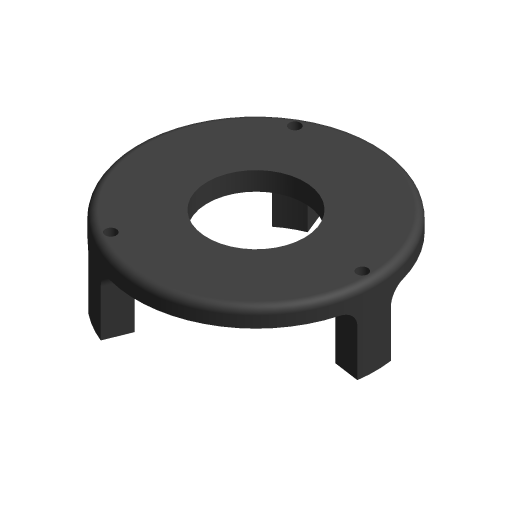
# Autodesk Inventor part: Engine retention
Saved by Autodesk Inventor 2024 (Build 280153000, 153)
## iProperties
Part Number: Engine retention
Material: Generic
Document SubType Name: Modeling
Designer: Jamie
Appearance: Default
Author: Jamie
Autodesk Inventor part; units mm, degrees
ref_plane "YZ Plane" through (0, 0, 0) normal (1, 0, 0) x (0, 1, 0)
ref_plane "XZ Plane" through (0, 0, 0) normal (0, 1, 0) x (-1, 0, 0)
ref_plane "XY Plane" through (0, 0, 0) normal (0, 0, 1) x (1, 0, 0)
sketch "Sketch1" plane through (0, 0, 0) normal (0, 1, 0) x (-1, 0, 0)
  circle A0 centre (0, 0) radius 25
  circle A1 centre (0, 0) radius 32
  dimension "d0" = 50
  dimension "d1" = 64
  constraints: 2 centre point, 2 coincident
  measures "d0" diameter of A0
  measures "d1" diameter of A1
extrude "Extrusion1" add sketch "Sketch1" along normal blind 16.5
sketch "Sketch2" plane through (0, 16.5, 0) normal (0, 1, 0) x (1, 0, 0)
  circle A0 centre (0, 0) radius 13
  circle A1 centre (0, 0) radius 32
  dimension "d4" = 26
  constraints: 2 centre point, 2 coincident
  measures "d4" diameter of A0
extrude "Extrusion2" add sketch "Sketch2" along normal blind 5
sketch "Sketch4" plane through (0, 0, 0) normal (0, -1, 0) x (1, 0, 0)
  circle A0 centre (28.5, 0) radius 1.5
  circle A1 centre (0, 0) radius 25 projected
  circle A2 centre (0, 0) radius 32 projected
  dimension "d7" = 3
  dimension "d9" = 28.5
  constraints: 1 centre point
  measures "d7" diameter of A0
  measures "d9" distance of A2.centre A0.centre
extrude "Extrusion3" cut sketch "Sketch4" against normal through all contours A0
pattern_circular "Circular Pattern1" count 3 over 360 about axis through (0, 0, 0) along (0, 1, 0) of "Extrusion3"
sketch "Sketch5" plane through (0, 0, 0) normal (0, -1, 0) x (1, 0, 0)
  line L0 (0, 0) -> (36.13577, -5.122389)
  line L1 (36.13577, -5.122389) -> (37.678755, -25.438365)
  line L2 (37.678755, -25.438365) -> (-15.629216, -38.816532)
  circle A0 centre (0, 0) radius 32
  line L3 (-15.629216, -38.816532) -> (0, 0)
  circle A1 centre (28.5, 0) radius 1.5
  circle A2 centre (-14.25, -24.681724) radius 1.5
  point P0 (-11.952112, -29.684121)
  point P1 (31.683259, -4.491228)
  dimension "d15" = 4
  dimension "d22" = 4
  constraints: 8 end point
  measures "d15" distance from line of A1.centre L0
  measures "d22" distance from line of A2.centre L3
extrude "Extrusion4" cut sketch "Sketch5" against normal blind 16.5 contours L0 A0 L3 picked at (20.515863, -5.328549)
pattern_circular "Circular Pattern2" count 3 over 360 about axis through (0, 16.5, 0) along (0, 1, 0) of "Extrusion4"
fillet "Fillet1" radius 4 6 edges at (28.2179, 16.5, -4) (-10.6448, 16.5, -26.4374) (-17.5731, 16.5, -22.4374) (-17.5731, 16.5, 22.4374) (-10.6448, 16.5, 26.4374) (28.2179, 16.5, 4)
fillet "Fillet2" radius 2 1 edges at (-32, 21.5, 0)
body "Solid1"
